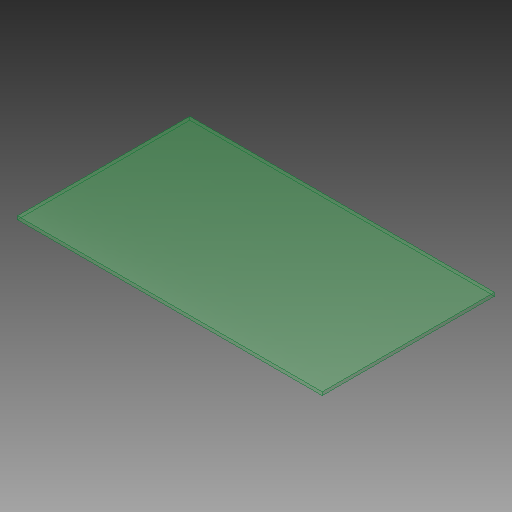
# Autodesk Inventor part: sb_bottom
Saved by Autodesk Inventor 2018.1 (Build 221171000, 171)
## iProperties
Created: 2017-08-17
Part Number: sb_bottom
Material: PVC-Piping
Document SubType Name: Modeling
Designer: Tom
Density: 1.4 g/cm^3
Appearance: Clear - Green 1
Author: Tom
Autodesk Inventor part; units mm, degrees
ref_plane "YZ Plane" through (0, 0, 0) normal (1, 0, 0) x (0, 1, 0)
ref_plane "XZ Plane" through (0, 0, 0) normal (0, 1, 0) x (-1, 0, 0)
ref_plane "XY Plane" through (0, 0, 0) normal (0, 0, 1) x (1, 0, 0)
sketch "Sketch1" plane through (0, 0, 0) normal (0, 1, 0) x (-1, 0, 0)
  line L0 (230, 130) -> (-230, 130)
  line L1 (-230, 130) -> (-230, -130)
  line L2 (-230, -130) -> (230, -130)
  line L3 (230, -130) -> (230, 130)
  line L4 (230, 130) -> (-230, -130) construction
  line L5 (-230, 130) -> (230, -130) construction
  point P0 (0, 0)
  dimension "d0" = 460
  dimension "d1" = 260
  constraints: 12 end point, 2 midpoint, 2 parallel, 1 horizontal, 1 perpendicular
  measures "d0" distance of L2.end L1.end
  measures "d1" distance of L1.end L0.end
extrude "Extrusion1" add sketch "Sketch1" along normal blind 5
equation "\"d0\" = boxw + 2 * pvct"
equation "\"d1\" = boxl + 2 * pvct"
equation "\"d2\" = pvct"
equation "\"solhole\" = 3"
equation "\"solholespacing\" = 16"
equation "\"ssolw\" = 63"
equation "\"bsoll\" = 126"
equation "\"bsolw\" = 91"
equation "\"bsolh\" = 126"
equation "\"tapl\" = 31"
equation "\"tl\" = 32"
equation "\"eloboww\" = 25"
equation "\"pvct\" = 5"
equation "\"boxh\" = 258"
equation "\"supporth\" = 15"
equation "\"play\" = 0.5"
equation "\"psuh\" = 85"
equation "\"arl\" = 102"
equation "\"pcbw\" = 76"
equation "\"pcbh\" = 46"
equation "\"arw\" = 54"
equation "\"pcbl\" = 86"
equation "\"screenl\" = 115"
equation "\"screenw\" = 197"
equation "\"seph\" = 105"
equation "\"diaetapeouter\" = 36"
equation "\"diaload\" = 16"
equation "\"diaphouter\" = 48"
equation "\"diapowerouter\" = 25"
equation "\"dialoadouter\" = 25"
equation "\"diaetape\" = 25"
equation "\"diaph\" = 32"
equation "\"distbubblewater\" = 82"
equation "\"distpumps\" = 75"
equation "\"diapower\" = 16"
equation "\"airoutinner\" = 28"
equation "\"airininner\" = 28"
equation "\"airoutouter\" = 39"
equation "\"pumpouter\" = 25"
equation "\"airinouter\" = 39"
equation "\"waterinner\" = 28"
equation "\"pumpinner\" = 16"
equation "\"waterouter\" = 39"
equation "\"boxw\" = 450"
equation "\"boxl\" = 250"
body "Solid1"
